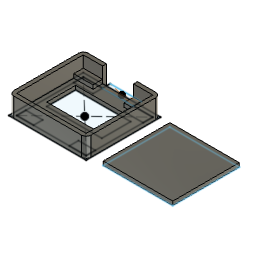
oled_cover (Autodesk Fusion 360 design; units mm, degrees)
Autodesk Fusion 360 part; units mm, degrees
sketch "Sketch1" plane through (0, 0, 0) normal (0, 0, 1) x (1, 0, 0)
  line L0 (14.45, -13.85) -> (-14.45, -13.85)
  line L1 (-14.45, -13.85) -> (-14.45, 13.85)
  line L2 (-14.45, 13.85) -> (14.45, 13.85)
  line L3 (14.45, 13.85) -> (14.45, -13.85)
  line L4 (14.45, -13.85) -> (-14.45, 13.85) construction
  line L5 (-14.45, -13.85) -> (14.45, 13.85) construction
  line L6 (-14.45, 13.85) -> (-6.45, 13.85)
  line L7 (-6.45, 13.85) -> (-6.45, 9.85)
  line L8 (-6.45, 9.85) -> (-14.45, 9.85)
  line L9 (-14.45, 9.85) -> (-14.45, 13.85)
  line L10 (14.45, 13.85) -> (6.45, 13.85)
  line L11 (6.45, 13.85) -> (6.45, 9.85)
  line L12 (6.45, 9.85) -> (14.45, 9.85)
  line L13 (14.45, 9.85) -> (14.45, 13.85)
  line L14 (-14.45, -13.85) -> (-7.45, -13.85)
  line L15 (-7.45, -13.85) -> (-7.45, -10.05)
  line L16 (-7.45, -10.05) -> (-14.45, -10.05)
  line L17 (-14.45, -10.05) -> (-14.45, -13.85)
  line L18 (14.45, -13.85) -> (7.45, -13.85)
  line L19 (7.45, -13.85) -> (7.45, -10.05)
  line L20 (7.45, -10.05) -> (14.45, -10.05)
  line L21 (14.45, -10.05) -> (14.45, -13.85)
  line L22 (-11.45, 7.65) -> (11.45, 7.65)
  line L23 (11.45, 7.65) -> (11.45, -4.35)
  line L24 (11.45, -4.35) -> (-11.45, -4.35)
  line L25 (-11.45, -4.35) -> (-11.45, 7.65)
  line L26 (16.05, -15.45) -> (-16.05, -15.45)
  line L27 (-16.05, -15.45) -> (-16.05, 15.45)
  line L28 (-16.05, 15.45) -> (16.05, 15.45)
  line L29 (16.05, 15.45) -> (16.05, -15.45)
  line L30 (6.45, 13.85) -> (-6.45, 13.85)
  line L31 (-6.45, 13.85) -> (-6.45, 17.05)
  line L32 (-6.45, 17.05) -> (6.45, 17.05)
  line L33 (6.45, 17.05) -> (6.45, 13.85)
  line L34 (6.45, 13.85) -> (-6.45, 17.05) construction
  line L35 (-6.45, 13.85) -> (6.45, 17.05) construction
  line L36 (21.55, -13.85) -> (21.55, 13.85)
  line L37 (50.45, -13.85) -> (21.55, -13.85)
  line L38 (50.45, 13.85) -> (50.45, -13.85)
  line L39 (21.55, 13.85) -> (50.45, 13.85)
  point P0 (0, 15.45)
  dimension "d1" = 28.9
  dimension "d2" = 27.7
  dimension "d3" = 8
  dimension "d4" = 4
  dimension "d5" = 8
  dimension "d6" = 4
  dimension "d7" = 7
  dimension "d8" = 3.8
  dimension "d9" = 7
  dimension "d10" = 3.8
  dimension "d11" = 22.9
  dimension "d12" = 12
  dimension "d13" = 6.2
  dimension "d14" = 3
  dimension "d15" = -1.6
  dimension "d16" = 12.9
  dimension "d23" = 28.9
  dimension "d24" = 27.7
  constraint horizontal L0
  constraint perpendicular L0 L1
  constraint parallel L0 L2
  constraint parallel L1 L3
  constraint coincident L4 origin
  constraint coincident L5 origin
  constraint horizontal L6
  constraint vertical L7
  constraint horizontal L8
  constraint vertical L9
  constraint horizontal L10
  constraint vertical L11
  constraint horizontal L12
  constraint vertical L13
  constraint horizontal L14
  constraint vertical L15
  constraint horizontal L16
  constraint vertical L17
  constraint horizontal L18
  constraint vertical L19
  constraint horizontal L20
  constraint vertical L21
  constraint horizontal L22
  constraint vertical L23
  constraint horizontal L24
  constraint vertical L25
  constraint horizontal L30
  constraint perpendicular L30 L31
  constraint parallel L30 L32
  constraint parallel L31 L33
  constraint coincident L34 P0
  constraint coincident L35 P0
  constraint midpoint L28 P0
  constraint horizontal L37
  constraint perpendicular L36 L37
  constraint parallel L37 L39
  constraint parallel L36 L38
  measures "d1" distance of L1.end L2.end
  measures "d2" distance of L0.end L1.end
  measures "d3" distance of L1.end L6.end
  measures "d4" distance of L1.end L8.end
  measures "d5" distance of L2.end L10.end
  measures "d6" distance of L2.end L12.end
  measures "d7" distance of L0.end L14.end
  measures "d8" distance of L0.end L16.end
  measures "d9" distance of L0.start L18.end
  measures "d10" distance of L0.start L20.end
  measures "d11" distance of L22.start L22.end
  measures "d12" distance of L22.start L24.end
  measures "d13" distance of L2 L22
  measures "d14" distance of L1 L25
  measures "d16" distance of L31.end L32.end
  measures "d23" distance of L36.end L38.start
  measures "d24" distance of L36.start L36.end
extrude "Extrude4" add sketch "Sketch1" along normal blind 1.6 contours L36 L37 L38 L39 makes body 1
extrude "Extrude3" add sketch "Sketch1" along normal blind 8 separate body contours L0 L1 L2 L3 L6 L9 L10 L13 L14 L17 L18 L21 L26 L27 L28 L29 L31 L33 makes body 2
extrude "Extrude2" add sketch "Sketch1" along normal blind 3.2 separate body contours L0 L3 L18 L19 L20 L21 | L0 L1 L14 L15 L16 L17 | L2 L3 L10 L11 L12 L13 | L1 L2 L6 L7 L8 L9 makes body 3 at (12.1167, -12.5833, 0) makes body 4 at (9.1167, 11.1833, 0) makes body 5 at (-9.7833, -12.5833, 0) makes body 6 at (-11.7833, 12.5167, 0)
extrude "Extrude1" add sketch "Sketch1" along normal blind 1.6 separate body contours L0 L1 L2 L3 L7 L8 L11 L12 L15 L16 L19 L20 L30 makes body 7
fillet "Fillet1" radius 2 4 edges at (-16.05, -15.45, 4) (16.05, -15.45, 4) (16.05, 15.45, 4) (-16.05, 15.45, 4) on bodies 2
